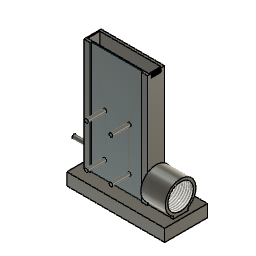
Finflow_beaker_new v6 (Autodesk Fusion 360 design; units mm, degrees)
Autodesk Fusion 360 part; units mm, degrees
sketch "Sketch1" plane through (0, 0, 0) normal (0, 0, 1) x (1, 0, 0)
  line L0 (0, 0) -> (52, 0)
  line L1 (52, 0) -> (52, 12)
  line L2 (52, 12) -> (0, 12)
  line L3 (0, 12) -> (0, 0)
  dimension "d1" = 52
  dimension "d2" = 12
  constraint horizontal L0
  constraint vertical L1
  constraint horizontal L2
  constraint vertical L3
  constraint coincident L0.start L3.end
  measures "d1" distance of L0.start L0.end
  measures "d2" distance of L0.start L2.end
extrude "Extrude1" add sketch "Sketch1" along normal blind 1 makes body 1
extrude "Extrude2" add 1 faces at (17.3333, 8, 1) along direction (0, 0, 1) blind 1 on bodies 1 bodies 1
sketch "Sketch2" plane through (0, 0, 2) normal (0, 0, 1) x (-1, 0, 0)
  line L0 (0, -12) -> (0, 0)
  line L1 (0, 0) -> (-52, 0)
  line L2 (-52, 0) -> (-52, -12)
  line L3 (-52, -12) -> (0, -12)
  line L4 (-1, -11) -> (-51, -11)
  line L5 (-51, -11) -> (-51, -1)
  line L6 (-51, -1) -> (-1, -1)
  line L7 (-1, -1) -> (-1, -11)
  dimension "d7" = 50
  dimension "d8" = 10
  constraint horizontal L4
  constraint vertical L5
  constraint horizontal L6
  constraint vertical L7
  measures "d7" distance of L4.start L4.end
  measures "d8" distance of L4.start L6.end
revolve "Revolve1" add sketch "Sketch2" angle 5 about axis through (51, 11, 2) along (0, 1, 0) contours L4 L5 L6 L7 bodies 1
sketch "Sketch3" plane through (52, 0, 0) normal (1, 0, 0) x (0, 1, 0)
  line L0 (0, 0) -> (12, 0)
  line L1 (12, 0) -> (12, 2)
  line L2 (12, 2) -> (0, 2)
  line L3 (0, 2) -> (0, 0)
  line L4 (0, 2) -> (12, 2)
  line L5 (12, 2) -> (12, 92)
  line L6 (12, 92) -> (0, 92)
  line L7 (0, 92) -> (0, 2)
  dimension "d10" = 12
  dimension "d11" = 90
  constraint horizontal L4
  constraint vertical L5
  constraint horizontal L6
  constraint vertical L7
  constraint coincident L2.end L3.start
  measures "d10" distance of L2.end L1.end
  measures "d11" distance of L2.end L6.end
extrude "Extrude3" add sketch "Sketch3" against normal blind 1 contours L2 L4 L5 L6 L7 bodies 1
sketch "Sketch4" plane through (0, 0, 0) normal (-1, 0, 0) x (0, -1, 0)
  line L0 (-12, 0) -> (0, 0)
  line L1 (0, 0) -> (0, 2)
  line L2 (0, 2) -> (-12, 2)
  line L3 (-12, 2) -> (-12, 0)
  line L4 (-12, 2) -> (0, 2)
  line L5 (0, 2) -> (0, 92)
  line L6 (0, 92) -> (-12, 92)
  line L7 (-12, 92) -> (-12, 2)
  dimension "d14" = 90
  constraint horizontal L4
  constraint vertical L5
  constraint horizontal L6
  constraint vertical L7
  constraint coincident L2.end L3.start
  measures "d14" distance of L2.end L6.end
extrude "Extrude4" add sketch "Sketch4" against normal blind 1 contours L2 L4 L5 L6 L7 bodies 1
sketch "Sketch5" plane through (0, 0, 0) normal (0, -1, 0) x (1, 0, 0)
  line L0 (0, 0) -> (52, 0)
  line L1 (52, 0) -> (52, 92)
  line L2 (52, 92) -> (51, 92)
  line L3 (51, 92) -> (51, 2)
  line L4 (51, 2) -> (1, 2)
  line L5 (1, 2) -> (1, 92)
  line L6 (1, 92) -> (0, 92)
  line L7 (0, 92) -> (0, 0)
  line L8 (1, 2) -> (51, 2)
  line L9 (51, 2) -> (51, 92)
  line L10 (51, 92) -> (1, 92)
  line L11 (1, 92) -> (1, 2)
  dimension "d17" = 50
  dimension "d18" = 90
  constraint horizontal L8
  constraint vertical L9
  constraint horizontal L10
  constraint vertical L11
  constraint coincident L4.end L5.start
  measures "d17" distance of L4.end L3.end
  measures "d18" distance of L4.end L5.end
extrude "Extrude5" add sketch "Sketch5" against normal blind 1 contours L3 L4 L5 L8 L9 L10 L11 bodies 1
sketch "Sketch6" plane through (0, 0, 0) normal (-1, 0, 0) x (0, -1, 0)
  line L0 (-12, 0) -> (0, 0)
  line L1 (0, 0) -> (0, 92)
  line L2 (0, 92) -> (-12, 92)
  line L3 (-12, 92) -> (-12, 0)
  circle A0 centre (-6, 8.7038) radius 1.75
  dimension "d21" = 3.5
  measures "d21" diameter of A0
extrude "Extrude6" add sketch "Sketch6" along normal blind 15 contours A0 bodies 1
sketch "Sketch7" plane through (-15, 0, 0) normal (-1, 0, 0) x (0, -1, 0)
  circle A0 centre (-6, 8.7038) radius 1.75
  circle A1 centre (-6, 8.7038) radius 1.15
  dimension "d24" = 2.3
  constraint concentric A0 A1
  measures "d24" diameter of A1
extrude "Extrude7" cut sketch "Sketch7" against normal blind 16 contours A1 bodies 1
sketch "Sketch8" plane through (0, 0, 0) normal (0, -1, 0) x (1, 0, 0)
  line L0 (0, 0) -> (52, 0)
  line L1 (52, 0) -> (52, 92)
  line L2 (52, 92) -> (0, 92)
  line L3 (0, 92) -> (0, 0)
  circle A0 centre (16, 14) radius 2
  dimension "d27" = 4
  measures "d27" diameter of A0
sketch "Sketch9" plane through (0, 0, 0) normal (0, -1, 0) x (1, 0, 0)
sketch "Sketch10" plane through (0, 0, 0) normal (0, -1, 0) x (1, 0, 0)
sketch "Sketch11" plane through (26, 0, 46) normal (0, -1, 0) x (1, 0, 0)
sketch "Sketch12" plane through (26, 0, 46) normal (0, -1, 0) x (1, 0, 0)
  circle A0 centre (10, -32) radius 2
extrude "Extrude8" add sketch "Sketch8" along normal blind 15 contours A0 bodies 1
extrude "Extrude9" add sketch "Sketch12" along normal blind 15 bodies 1
sketch "Sketch13" plane through (0, 0, 0) normal (0, -1, 0) x (1, 0, 0)
  line L0 (0, 0) -> (52, 0)
  line L1 (52, 0) -> (52, 92)
  line L2 (52, 92) -> (0, 92)
  line L3 (0, 92) -> (0, 0)
sketch "Sketch14" plane through (0, 0, 0) normal (0, -1, 0) x (1, 0, 0)
  circle A0 centre (16, 49) radius 2
  circle A1 centre (36, 49) radius 2
sketch "Sketch15" plane through (0, 0, 0) normal (0, -1, 0) x (1, 0, 0)
extrude "Extrude10" add sketch "Sketch14" along normal blind 15 contours A0 bodies 1
sketch "Sketch16" plane through (0, 0, 0) normal (0, -1, 0) x (1, 0, 0)
  circle A0 centre (36, 49) radius 2
  dimension "d34" = 4
  measures "d34" diameter of A0
extrude "Extrude11" add sketch "Sketch16" along normal blind 15 bodies 1
sketch "Sketch17" plane through (52, 0, 0) normal (1, 0, 0) x (0, 1, 0)
  line L0 (0, 0) -> (12, 0)
  line L1 (12, 0) -> (12, 92)
  line L2 (12, 92) -> (0, 92)
  line L3 (0, 92) -> (0, 0)
  line L4 (2, 91) -> (10, 91)
  line L5 (10, 91) -> (10, 89)
  line L6 (10, 89) -> (2, 89)
  line L7 (2, 89) -> (2, 91)
  dimension "d37" = 8
  constraint horizontal L4
  constraint vertical L5
  constraint horizontal L6
  constraint vertical L7
  measures "d37" distance of L4.start L4.end
extrude "Extrude12" cut sketch "Sketch17" against normal blind 1 contours L4 L5 L6 L7 bodies 1
sketch "Sketch18" plane through (52, 0, 0) normal (1, 0, 0) x (0, 1, 0)
  line L0 (10, 91) -> (10, 89)
  line L1 (10, 89) -> (2, 89)
  line L2 (2, 89) -> (2, 91)
  line L3 (2, 91) -> (10, 91)
  line L4 (0, 0) -> (12, 0)
  line L5 (12, 0) -> (12, 92)
  line L6 (12, 92) -> (0, 92)
  line L7 (0, 92) -> (0, 0)
  circle A0 centre (6, 13) radius 12.5
  dimension "d40" = 25
  measures "d40" diameter of A0
extrude "Extrude13" add sketch "Sketch18" along normal blind 20 contours L4 L5 L7 A0 | L7 A0 | L5 L7 A0 | L5 A0 bodies 1
sketch "Sketch19" plane through (72, 0, 0) normal (1, 0, 0) x (0, 1, 0)
  arc A0 (12, 2.0341) -> (0, 2.0341) centre (6, 13) ccw
  line L0 (0, 2.0341) -> (0, 0)
  line L1 (0, 0) -> (12, 0)
  line L2 (12, 0) -> (12, 2.0341)
  circle A1 centre (6, 13) radius 9.575
  dimension "d43" = 19.15
  constraint concentric A0 A1
  measures "d43" diameter of A1
extrude "Extrude14" cut sketch "Sketch19" against normal blind 19 contours A1 bodies 1
sketch "Sketch20" plane through (53, 0, 0) normal (1, 0, 0) x (0, 1, 0)
  circle A0 centre (6, 13) radius 9.575
  circle A1 centre (6, 9) radius 4
  dimension "d46" = 8
  measures "d46" diameter of A1
revolve "Revolve2" cut 1 faces at (34.3968, 4.3333, 3.4526) angle 5 about axis through (51, 11, 2) along (0, -1, 0) on bodies 1 bodies 1
delete_face "DeleteFace1" 1 faces at (-10, 4.2587, 8.5295) on bodies 1
extrude "Extrude15" add 1 faces at (34.3333, 4.3333, 2) along direction (0, 0, 1) blind 3 on bodies 1 bodies 1
sketch "Sketch21" plane through (0, 0, 5) normal (0, 0, 1) x (-1, 0, 0)
  line L0 (-1, -12) -> (-1, -1)
  line L1 (-1, -1) -> (-51, -1)
  line L2 (-51, -1) -> (-51, -12)
  line L3 (-51, -12) -> (-1, -12)
  line L4 (-1, -1) -> (-51, -1)
  line L5 (-51, -1) -> (-51, -11)
  line L6 (-51, -11) -> (-1, -11)
  line L7 (-1, -11) -> (-1, -1)
  dimension "d50" = 10
  constraint horizontal L4
  constraint vertical L5
  constraint horizontal L6
  constraint vertical L7
  constraint coincident L0.end L1.start
  measures "d50" distance of L0.end L6.end
revolve "Revolve3" add sketch "Sketch21" angle 5 about axis through (51, 1, 5) along (0, 1, 0) contours L0 L1 L2 L4 L5 L6 L7 bodies 1
cylinder "CylinderPrimitive1" add diameter 2.3 height -1 placed x (0, 0, 1) y (0, 1, 0) z (-1, 0, 0) at (0, 6, 8.7038) bodies 1
extrude "Extrude16" cut sketch "Sketch20" against normal blind 2 contours A1 bodies 1
sketch "Sketch23" plane through (0, 0, 0) normal (-1, 0, 0) x (0, -1, 0)
  line L0 (-12, 0) -> (0, 0)
  line L1 (0, 0) -> (0, 92)
  line L2 (0, 92) -> (-12, 92)
  line L3 (-12, 92) -> (-12, 0)
  circle A0 centre (-6, 12) radius 1.75
  dimension "d56" = 3.5
  measures "d56" diameter of A0
extrude "Extrude17" add sketch "Sketch23" along normal blind 15 contours A0 bodies 1
sketch "Sketch24" plane through (-15, 0, 0) normal (-1, 0, 0) x (0, -1, 0)
  circle A0 centre (-6, 12) radius 1.75
  circle A1 centre (-6, 12) radius 1.2
  dimension "d59" = 2.4
  constraint concentric A0 A1
  measures "d59" diameter of A1
extrude "Extrude18" cut sketch "Sketch24" against normal blind 17 contours A1 bodies 1
sketch "Sketch25" plane through (0, 12, 0) normal (0, 1, 0) x (-1, 0, 0)
  line L0 (-72, 0) -> (0, 0)
  line L1 (0, 0) -> (0, 92)
  line L2 (0, 92) -> (-1, 92)
  line L3 (-1, 92) -> (-1, 5)
  line L4 (-1, 5) -> (-51, 5)
  line L5 (-51, 5) -> (-51, 92)
  line L6 (-51, 92) -> (-52, 92)
  line L7 (-52, 92) -> (-52, 23.9659)
  line L8 (-52, 23.9659) -> (-52, 2.0341)
  line L9 (-52, 2.0341) -> (-72, 2.0341)
  line L10 (-72, 2.0341) -> (-72, 0)
  line L11 (-51, 5) -> (-1, 5)
  line L12 (-1, 5) -> (-1, 92)
  line L13 (-1, 92) -> (-51, 92)
  line L14 (-51, 92) -> (-51, 5)
  constraint horizontal L11
  constraint vertical L12
  constraint horizontal L13
  constraint vertical L14
  constraint coincident L2 L3.start
  constraint coincident L3 L2.end
  constraint coincident L4.end L5.start
extrude "Extrude19" add sketch "Sketch25" against normal blind 1 contours L3 L4 L5 L11 L12 L13 L14 bodies 1
sketch "Sketch26" plane through (0, 12, 0) normal (0, 1, 0) x (-1, 0, 0)
  line L0 (-72, 0) -> (0, 0)
  line L1 (0, 0) -> (0, 92)
  line L2 (0, 92) -> (-52, 92)
  line L3 (-52, 92) -> (-52, 23.9659)
  line L4 (-52, 23.9659) -> (-52, 2.0341)
  line L5 (-52, 2.0341) -> (-72, 2.0341)
  line L6 (-72, 2.0341) -> (-72, 0)
  line L7 (-39, 18.5) -> (-13, 18.5)
  line L8 (-13, 18.5) -> (-13, 44.5)
  line L9 (-13, 44.5) -> (-39, 44.5)
  line L10 (-39, 44.5) -> (-39, 18.5)
  dimension "d64" = 26
  dimension "d65" = 26
  constraint horizontal L7
  constraint vertical L8
  constraint horizontal L9
  constraint vertical L10
  measures "d64" distance of L7.start L7.end
  measures "d65" distance of L7.start L9.end
extrude "Extrude20" add sketch "Sketch26" along normal blind 3 contours L7 L8 L9 L10 bodies 1
sketch "Sketch27" plane through (0, 15, 0) normal (0, 1, 0) x (-1, 0, 0)
  line L0 (-39, 44.5) -> (-39, 18.5)
  line L1 (-39, 18.5) -> (-13, 18.5)
  line L2 (-13, 18.5) -> (-13, 44.5)
  line L3 (-13, 44.5) -> (-39, 44.5)
  line L4 (-38, 19.5) -> (-14, 19.5)
  line L5 (-14, 19.5) -> (-14, 43.5)
  line L6 (-14, 43.5) -> (-38, 43.5)
  line L7 (-38, 43.5) -> (-38, 19.5)
  dimension "d68" = 24
  dimension "d69" = 24
  constraint horizontal L4
  constraint vertical L5
  constraint horizontal L6
  constraint vertical L7
  measures "d68" distance of L4.start L4.end
  measures "d69" distance of L4.start L6.end
extrude "Extrude21" cut sketch "Sketch27" against normal blind 3 contours L4 L5 L6 L7 bodies 1
sketch "Sketch28" plane through (0, 12, 0) normal (0, 1, 0) x (-1, 0, 0)
  line L0 (-38, 43.5) -> (-38, 19.5)
  line L1 (-38, 19.5) -> (-14, 19.5)
  line L2 (-14, 19.5) -> (-14, 43.5)
  line L3 (-14, 43.5) -> (-38, 43.5)
  line L4 (-37, 42.5) -> (-15, 42.5)
  line L5 (-15, 42.5) -> (-15, 20.5)
  line L6 (-15, 20.5) -> (-37, 20.5)
  line L7 (-37, 20.5) -> (-37, 42.5)
  dimension "d72" = 22
  dimension "d73" = 22
  constraint horizontal L4
  constraint vertical L5
  constraint horizontal L6
  constraint vertical L7
  measures "d72" distance of L4.start L4.end
  measures "d73" distance of L4.start L6.end
extrude "Extrude22" add sketch "Sketch28" along normal blind 3 contours L4 L5 L6 L7 bodies 1
sketch "Sketch29" plane through (0, 15, 0) normal (0, 1, 0) x (-1, 0, 0)
  line L0 (-37, 20.5) -> (-15, 20.5)
  line L1 (-15, 20.5) -> (-15, 42.5)
  line L2 (-15, 42.5) -> (-37, 42.5)
  line L3 (-37, 42.5) -> (-37, 20.5)
  line L4 (-36, 41.5) -> (-16, 41.5)
  line L5 (-16, 41.5) -> (-16, 21.5)
  line L6 (-16, 21.5) -> (-36, 21.5)
  line L7 (-36, 21.5) -> (-36, 41.5)
  dimension "d76" = 20
  dimension "d77" = 20
  constraint horizontal L4
  constraint vertical L5
  constraint horizontal L6
  constraint vertical L7
  measures "d76" distance of L4.start L4.end
  measures "d77" distance of L4.start L6.end
extrude "Extrude23" cut sketch "Sketch29" against normal blind 3 contours L4 L5 L6 L7 bodies 1
sketch "Sketch30" plane through (0, 0, 0) normal (0, 0, -1) x (1, 0, 0)
  line L0 (0, 0) -> (0, -12)
  line L1 (0, -12) -> (72, -12)
  line L2 (72, -12) -> (72, 0)
  line L3 (72, 0) -> (0, 0)
  line L4 (-5, 10) -> (75, 10)
  line L5 (75, 10) -> (75, -25)
  line L6 (75, -25) -> (-5, -25)
  line L7 (-5, -25) -> (-5, 10)
  constraint horizontal L4
  constraint vertical L5
  constraint horizontal L6
  constraint vertical L7
extrude "Extrude24" add sketch "Sketch30" along normal blind 10 separate body makes body 2
extrude "Extrude25" add 1 faces at (48, 8, 0) along direction (0, 0, -1) blind 10 on bodies 1 bodies 1 2
sketch "Sketch31" plane through (26, 0, 46) normal (0, -1, 0) x (1, 0, 0)
  line L0 (-26, 46) -> (-21, 46)
  line L1 (-21, 46) -> (-21, -46)
  line L2 (-21, -46) -> (-26, -46)
  line L3 (-26, -46) -> (-26, 46)
  dimension "d84" = 5
  dimension "d85" = 92
  constraint horizontal L0
  constraint vertical L1
  constraint horizontal L2
  constraint vertical L3
  measures "d84" distance of L0.start L0.end
  measures "d85" distance of L0.start L2.end
extrude "Extrude26" add sketch "Sketch31" along normal blind 1 bodies 1
sketch "Sketch32" plane through (26, 0, 46) normal (0, -1, 0) x (1, 0, 0)
  line L0 (26, 46) -> (21, 46)
  line L1 (21, 46) -> (21, -46)
  line L2 (21, -46) -> (26, -46)
  line L3 (26, -46) -> (26, 46)
  dimension "d88" = 5
  dimension "d89" = 92
  constraint horizontal L0
  constraint vertical L1
  constraint horizontal L2
  constraint vertical L3
  measures "d88" distance of L0.start L0.end
  measures "d89" distance of L0.start L2.end
extrude "Extrude27" add sketch "Sketch32" along normal blind 1 bodies 1
sketch "Sketch33" plane through (0, 12, 0) normal (0, 1, 0) x (-1, 0, 0)
  line L0 (-39, 44.5) -> (-13, 44.5)
  line L1 (-13, 44.5) -> (-13, 18.5)
  line L2 (-13, 18.5) -> (-39, 18.5)
  line L3 (-39, 18.5) -> (-39, 44.5)
  line L4 (-72, 0) -> (0, 0)
  line L5 (0, 0) -> (0, 92)
  line L6 (0, 92) -> (-52, 92)
  line L7 (-52, 92) -> (-52, 23.9659)
  line L8 (-52, 23.9659) -> (-52, 2.0341)
  line L9 (-52, 2.0341) -> (-72, 2.0341)
  line L10 (-72, 2.0341) -> (-72, 0)
  line L11 (0, 92) -> (-5, 92)
  line L12 (-5, 92) -> (-5, 0)
  line L13 (-5, 0) -> (0, 0)
  line L14 (0, 0) -> (0, 92)
  dimension "d92" = 5
  dimension "d93" = 92
  constraint horizontal L11
  constraint vertical L12
  constraint horizontal L13
  constraint vertical L14
  constraint coincident L5.end L6.start
  measures "d92" distance of L5.end L11.end
  measures "d93" distance of L5.end L4.end
extrude "Extrude28" add sketch "Sketch33" along normal blind 1 contours L4 L5 L6 L11 L12 L13 L14 bodies 1
sketch "Sketch34" plane through (0, 12, 0) normal (0, 1, 0) x (-1, 0, 0)
  line L0 (-5, 0) -> (-5, 92)
  line L1 (-5, 92) -> (-52, 92)
  line L2 (-52, 92) -> (-52, 23.9659)
  line L3 (-52, 23.9659) -> (-52, 2.0341)
  line L4 (-52, 2.0341) -> (-72, 2.0341)
  line L5 (-72, 2.0341) -> (-72, 0)
  line L6 (-72, 0) -> (-5, 0)
  line L7 (-39, 44.5) -> (-13, 44.5)
  line L8 (-13, 44.5) -> (-13, 18.5)
  line L9 (-13, 18.5) -> (-39, 18.5)
  line L10 (-39, 18.5) -> (-39, 44.5)
  line L11 (-52, 92) -> (-47, 92)
  line L12 (-47, 92) -> (-47, 0)
  line L13 (-47, 0) -> (-52, 0)
  line L14 (-52, 0) -> (-52, 92)
  dimension "d96" = 5
  dimension "d97" = 92
  constraint horizontal L11
  constraint vertical L12
  constraint horizontal L13
  constraint vertical L14
  constraint coincident L1.end L2.start
  measures "d96" distance of L1.end L11.end
  measures "d97" distance of L1.end L13.end
extrude "Extrude29" add sketch "Sketch34" along normal blind 1 contours L1 L2 L3 L6 L11 L12 L13 L14 bodies 1
sketch "Sketch35" plane through (0, 12, 0) normal (0, 1, 0) x (-1, 0, 0)
  line L0 (-47, 92) -> (-47, 0)
  line L1 (-47, 0) -> (-5, 0)
  line L2 (-5, 0) -> (-5, 92)
  line L3 (-5, 92) -> (-47, 92)
  line L4 (-39, 44.5) -> (-13, 44.5)
  line L5 (-13, 44.5) -> (-13, 18.5)
  line L6 (-13, 18.5) -> (-39, 18.5)
  line L7 (-39, 18.5) -> (-39, 44.5)
  line L8 (-5, 0) -> (-47, 0)
  line L9 (-47, 0) -> (-47, 5)
  line L10 (-47, 5) -> (-5, 5)
  line L11 (-5, 5) -> (-5, 0)
  dimension "d100" = 42
  constraint horizontal L8
  constraint vertical L9
  constraint horizontal L10
  constraint vertical L11
  constraint coincident L1.end L2.start
  measures "d100" distance of L1.end L0.end
extrude "Extrude30" add sketch "Sketch35" along normal blind 1 contours L0 L1 L2 L8 L9 L10 L11 bodies 1
sketch "Sketch36" plane through (0, 12, 0) normal (0, 1, 0) x (-1, 0, 0)
  line L0 (-47, 5) -> (-5, 5)
  line L1 (-5, 5) -> (-5, 92)
  line L2 (-5, 92) -> (-47, 92)
  line L3 (-47, 92) -> (-47, 5)
  line L4 (-39, 44.5) -> (-13, 44.5)
  line L5 (-13, 44.5) -> (-13, 18.5)
  line L6 (-13, 18.5) -> (-39, 18.5)
  line L7 (-39, 18.5) -> (-39, 44.5)
  line L8 (-47, 92) -> (-5, 92)
  line L9 (-5, 92) -> (-5, 87)
  line L10 (-5, 87) -> (-47, 87)
  line L11 (-47, 87) -> (-47, 92)
  dimension "d103" = 42
  constraint horizontal L8
  constraint vertical L9
  constraint horizontal L10
  constraint vertical L11
  constraint coincident L2.end L3.start
  measures "d103" distance of L2.end L1.end
extrude "Extrude31" add sketch "Sketch36" along normal blind 1 contours L1 L2 L3 L8 L9 L10 L11 bodies 1
thread "Thread1" "ISO Pipe Threads 20.955 G20.955x1.814" major diameter 20.955 minor diameter 18.9015 pitch 1.8143 angle 55 resizes the face on face at (59.3333, 15.5274, 12.0466) on bodies 1
thread "Thread2" "ISO Pipe Threads 22.911 G22.911x1.814" major diameter 22.911 minor diameter 20.8575 pitch 1.8143 angle 55 resizes the face on face at (59.3333, 15.4038, 12.059) on bodies 1
move_face "MoveFace1" by (-1, 0, 0) 1 faces at (13, 13, 27.1667) on bodies 1
move_face "MoveFace2" by (-1, 0, 0) 1 faces at (14, 14, 27.5) on bodies 1
move_face "MoveFace3" by (0, 0, 1) 1 faces at (21, 14, 44.5) on bodies 1
move_face "MoveFace4" by (0, 0, 1) 1 faces at (21.3333, 13, 43.5) on bodies 1
move_face "MoveFace5" by (1, 0, 0) 1 faces at (39, 14, 36.5) on bodies 1
move_face "MoveFace6" by (1, 0, 0) 1 faces at (38, 13, 27.8333) on bodies 1
move_face "MoveFace7" by (0, 0, -1) 1 faces at (21.3333, 13, 18.5) on bodies 1
move_face "MoveFace8" by (0, 0, -1) 1 faces at (21.6667, 13, 19.5) on bodies 1
sketch "Sketch37" plane through (0, 0, 0) normal (0, -1, 0) x (1, 0, 0)
sketch "Sketch38" plane through (0, 0, 0) normal (0, -1, 0) x (1, 0, 0)
delete_face "DeleteFace2" 1 faces at (36.5417, -10, 15.9252) on bodies 1
sketch "Sketch39" plane through (0, 0, 0) normal (0, -1, 0) x (1, 0, 0)
  circle A0 centre (36, 14) radius 1.5
  dimension "d106" = 3
  measures "d106" diameter of A0
extrude "Extrude32" add sketch "Sketch39" along normal blind 15 bodies 1
delete_face "DeleteFace3" 2 faces at (15.8462, -15, 14.5774) (17.9975, -10, 14.0997) on bodies 1
delete_face "DeleteFace4" 2 faces at (35.9501, -10, 50.9994) (35.363, -15, 48.8035) on bodies 1
delete_face "DeleteFace5" 2 faces at (17.7564, -10, 49.9565) (16.6081, -15, 48.6114) on bodies 1
sketch "Sketch40" plane through (0, 0, 0) normal (0, -1, 0) x (1, 0, 0)
  circle A0 centre (16, 14) radius 1.5
  dimension "d109" = 3
  measures "d109" diameter of A0
sketch "Sketch41" plane through (0, 0, 0) normal (0, -1, 0) x (1, 0, 0)
  circle A0 centre (16, 49) radius 1.5
  circle A1 centre (36, 49) radius 1.5
  dimension "d110" = 3
  dimension "d111" = 3
  measures "d110" diameter of A0
  measures "d111" diameter of A1
extrude "Extrude33" add sketch "Sketch40" along normal blind 15 bodies 1
extrude "Extrude34" add sketch "Sketch41" along normal blind 15 contours A0 bodies 1
sketch "Sketch42" plane through (0, 0, 0) normal (0, -1, 0) x (1, 0, 0)
  circle A0 centre (36, 49) radius 1.5
  dimension "d116" = 3
  measures "d116" diameter of A0
extrude "Extrude35" add sketch "Sketch42" along normal blind 15 bodies 1
